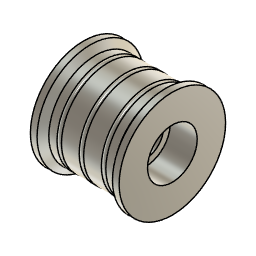
middle_pulley v3 (Autodesk Fusion 360 design; units mm, degrees)
Autodesk Fusion 360 part; units mm, degrees
sketch "Sketch1" plane through (0, 0, 0) normal (0, 1, 0) x (1, 0, 0)
  line L0 (0, 0) -> (10, 0)
  line L1 (10, 0) -> (10, -10.5)
  line L2 (10, -10.5) -> (0, -10.5)
  line L3 (0, -10.5) -> (0, 0)
  circle A0 centre (0, -10.5) radius 0.5
  circle A1 centre (5, -10.5) radius 0.5
  line L4 (10, -10.5) -> (10, -12)
  line L5 (10, -12) -> (8.5, -12)
  line L6 (8.5, -12) -> (7.355, -10.5)
  dimension "d1" = 10
  dimension "d2" = 10.5
  dimension "d3" = 1
  dimension "d4" = 1
  dimension "d5" = 5
  dimension "d6" = 1.5
  dimension "d7" = 1.5
  constraint horizontal L0
  constraint vertical L1
  constraint horizontal L2
  constraint vertical L3
  constraint coincident L0.start L3.end
  constraint coincident L2.end L3.start
  constraint coincident L2 A1.centre
  constraint perpendicular L2 L4
  constraint perpendicular L4 L5
  constraint coincident L2 L6.end
  measures "d1" distance of L0.start L0.end
  measures "d2" distance of L0.start L2.end
  measures "d3" diameter of A0
  measures "d4" diameter of A1
  measures "d5" distance of L2.end A1.centre
  measures "d6" distance of L1.end L4.end
  measures "d7" distance of L4.end L5.end
revolve "Revolve1" add sketch "Sketch1" angle 360 about axis through (0, 0, 0) along (1, 0, 0) contours L0 L1 L2 L3 A0 A1 | L2 L4 L5 L6
mirror "Mirror1" about plane through (0, 0, 0) normal (1, 0, 0) of bodies 1 merged
hole "Hole1" at (10, 0, 0) direction (-1, 0, 0) diameter 11.2 depth 20 tip angle 180
sketch "Sketch2" plane through (0, 0, 0) normal (0, 1, 0) x (1, 0, 0)
  line L0 (3.9329, -4.1) -> (1.9329, -4.1)
  line L1 (1.9329, -4.1) -> (1.9329, -5.6)
  line L2 (1.9329, -5.6) -> (3.9329, -5.6)
  line L3 (3.9329, -5.6) -> (3.9329, -4.1)
  line L4 (0, 0) -> (0, -6)
  line L5 (-1.9329, -5.6) -> (-3.9329, -5.6)
  line L6 (-3.9329, -5.6) -> (-3.9329, -4.1)
  line L7 (-3.9329, -4.1) -> (-1.9329, -4.1)
  line L8 (-1.9329, -4.1) -> (-1.9329, -5.6)
  point P0 (9.0329, -0.6479)
  point P1 (-10, 0)
  dimension "d14" = 2
  dimension "d15" = 1.5
  dimension "d16" = 5.1
  dimension "d18" = 5.6
  constraint horizontal L0
  constraint vertical L1
  constraint horizontal L2
  constraint vertical L3
  constraint coincident L4.start origin
  constraint vertical L4
  constraint symmetric L0.start L4 L6.end
  constraint symmetric L0.end L4 L7.end
  constraint symmetric L1.end L4 L5.start
  constraint symmetric L2.end L4 L5.end
  measures "d14" distance of L0.start L0.end
  measures "d15" distance of L0.start L2.end
  measures "d16" distance of L3 P0
  measures "d18" distance of L4.start L2
revolve "Revolve2" add sketch "Sketch2" angle 360 about axis through (1.75, 0, 0) along (1, 0, 0)
